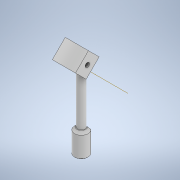
# Autodesk Inventor part: endoscope_holder_2
Saved by Autodesk Inventor 2022 (Build 260153000, 153)
## iProperties
Created: 2021-07-04
Part Number: endoscope_holder_2
Material: Generic
Document SubType Name: Modeling
Designer: dsdan
Density: 1 g/cm^3
Appearance: Default
Author: dsdan
Autodesk Inventor part; units mm, degrees
ref_plane "YZ Plane" through (0, 0, 0) normal (1, 0, 0) x (0, 1, 0)
ref_plane "XZ Plane" through (0, 0, 0) normal (0, 1, 0) x (-1, 0, 0)
ref_plane "XY Plane" through (0, 0, 0) normal (0, 0, 1) x (1, 0, 0)
sketch "Sketch1" plane through (0, 0, 0) normal (0, 1, 0) x (-1, 0, 0)
  circle A0 centre (0, 0) radius 3
  dimension "d0" = 6
  constraints: 1 centre point, 1 coincident
  measures "d0" diameter of A0
extrude "Extrusion1" add sketch "Sketch1" against normal blind 45
sketch "Sketch2" plane through (0, 0, 0) normal (1, 0, 0) x (0, 1, 0)
  line L0 (-45, 3) -> (-45, -3) projected
  line L1 (-43, 0) -> (-45, 0)
  line L2 (-45, 0) -> (-45, 3.55)
  line L3 (-43, 5.55) -> (-43, 0)
  line L4 (-43, 5.55) -> (-62, 5.55)
  line L5 (-62, 5.55) -> (-62, 3.55)
  line L6 (-62, 3.55) -> (-45, 3.55)
  line L7 (-45, 0) -> (-111.5, 0)
  point P0 (0, 0)
  dimension "d3" = 7.1
  dimension "d5" = 17
  dimension "d6" = 2
  dimension "d38" = 2
  constraints: 14 end point, 3 horizontal, 2 parallel, 2 perpendicular, 1 collinear, 1 midpoint, 1 point on line
  measures "d3" diameter of L6 L7
  measures "d5" distance between parallel lines of L2 L5
  measures "d6" distance between parallel lines of L3 L2
  measures "d38" distance between parallel lines of L6 L4
revolve "Revolution1" add sketch "Sketch2" angle 280 mid plane about axis through (0, -45, 0) along (0, -1, 0)
ref_plane "Work Plane3" through (0, 0, 0) normal (0, -0.7071068, 0.7071068) x (1, 0, 0)
sketch "Sketch8" plane through (0, 0, 0) normal (0, -0.7071068, 0.7071068) x (1, 0, 0)
  circle A0 centre (0, 9) radius 6.35
  circle A1 centre (0, 9) radius 11.35
  line L0 (-9.5, 2.7893) -> (-9.5, 15.2107)
  line L1 (9.5, 2.7893) -> (9.5, 15.2107)
  point P0 (0, 0)
  dimension "d44" = 12.7
  dimension "d45" = 5
  dimension "d46" = 19
  constraints: 4 end point, 4 point on circle, 2 centre point, 2 horizontal alignment, 1 coincident, 1 parallel, 1 vertical alignment
  measures "d44" diameter of A0
  measures "d45" radial gap between concentric circles of A1 A0
  measures "d46" distance between parallel lines of L0 L1
extrude "Extrusion8" add sketch "Sketch8" along normal blind 5 and the other way blind 10 contours L1 A1 L0
sketch "Sketch3" plane through (0, -45, 0) normal (0, -1, 0) x (1, 0, 0)
  circle A0 centre (0, 0) radius 1.2
  line L0 (1.2, 0) -> (-1.2, 0)
  line L1 (-1.2, 0) -> (-1.2, -21.8587)
  line L2 (-1.2, -21.8587) -> (1.2, -21.8587)
  line L3 (1.2, -21.8587) -> (1.2, 0)
  point P0 (-1.2, 0)
  point P1 (-1.2, 0)
  dimension "d11" = 2.4
  constraints: 8 end point, 2 parallel, 2 vertical, 1 coincident, 1 horizontal, 1 perpendicular, 3 other
extrude "Extrusion7" cut sketch "Sketch3" against normal up to surface round surface about axis through (0, 6.364, 6.364) along (0, -0.7071068, 0.7071068) radius 11.35 far side no
chamfer "Chamfer3" distance 0.4 angle 45 2 edges at (0, -62, 5.55) (0, -62, 3.55)
chamfer "Chamfer2" distance 2 angle 45 1 edges at (0, -43, 5.55)
chamfer "Chamfer5" distance 2 distance2 5 1 edges at (0, -45, 3.55) measured on face at (0, -45, 3.05)
fillet "Fillet2" radius 2 3 edges at (2.9902, -2.5146, -0.2418) (-2.6473, -1.4694, -1.4112) (-2.8041, -3.8921, 1.0663)
sketch "Sketch9" plane through (9.5, 7.22, 14.2911) normal (1, 0, 0) x (0, -0.7071068, -0.7071068)
  circle A0 centre (6.2107, 7.5) radius 1.8
  line L0 (12.4214, 15) -> (12.4214, 0) projected
  line L1 (12.4214, 0) -> (0, 0) projected
  point P0 (15.2107, 5)
  point P1 (12.4214, 7.5)
  point P2 (6.2107, 0)
  dimension "d53" = 3.6
  constraints: 2 midpoint, 1 centre point, 1 horizontal alignment, 1 vertical alignment
  measures "d53" diameter of A0
extrude "Extrusion9" cut sketch "Sketch9" against normal up to surface round surface about axis through (0, 6.364, 6.364) along (0, -0.7071068, 0.7071068) radius 6.35 far side no
body "Solid1"
